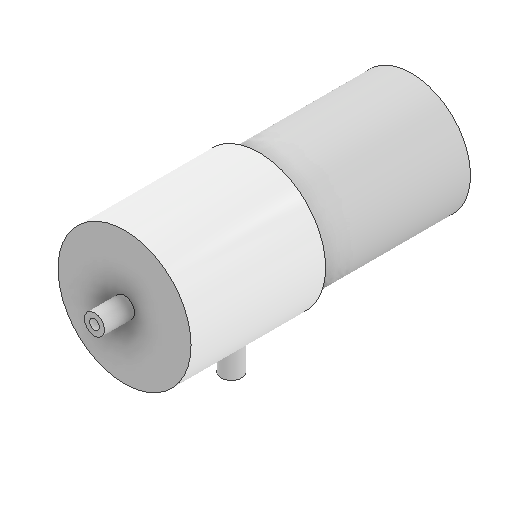
# Autodesk Inventor part: Adafruit_1528_4699_ND
Saved by Autodesk Inventor 2026.2 (Build 302298010, 298A)
## iProperties
Created: 2026-01-21
Part Number: Adafruit_1528_4699_ND
Material: Generic
Document SubType Name: Modeling
Designer: vckot
Density: 1 g/cm^3
Appearance: Default
Author: vckot
Autodesk Inventor part; units mm, degrees
ref_plane "XY Plane" through (0, 0, 0) normal (0, 0, 1) x (1, 0, 0)
sketch "Sketch1" plane through (0, 0, 0) normal (0, 0, 1) x (1, 0, 0)
  circle A0 centre (0, 0) radius 13.5
  circle A1 centre (0, 0) radius 2.05
  circle A2 centre (0, 0) radius 12
  circle A3 centre (0, 0) radius 1
  dimension "d0" = 27
  dimension "d3" = 4.1
  dimension "d6" = 24
  dimension "d20" = 2
  constraints: 4 centre point, 4 coincident
  measures "d0" diameter of A0
  measures "d3" diameter of A1
  measures "d6" diameter of A2
  measures "d20" diameter of A3
extrude "Extrusion1" add sketch "Sketch1" against normal blind 27.3 contours A0 | A1 | A2 | A3
extrude "Extrusion2" add sketch "Sketch1" along normal blind 6.1 contours A1 | A3
extrude "Extrusion3" add sketch "Sketch1" against normal blind 58.2 contours A1 | A2 | A3
ref_plane "Work Plane1" through (0, -13.5, 0) normal (0, 1, 0) x (-1, 0, 0)
sketch "Sketch2" plane through (0, -13.5, 0) normal (0, 1, 0) x (-1, 0, 0)
  circle A0 centre (0, -21.675) radius 2.875
  circle A1 centre (0, -21.675) radius 2.125
  line L0 (13.5, 0) -> (-13.5, 0) projected
  circle A2 centre (0, -21.675) radius 1
  point P0 (0, 0)
  dimension "d10" = 5.75
  dimension "d11" = 21.675
  dimension "d12" = 4.25
  dimension "d17" = 2
  constraints: 3 centre point, 2 coincident
  measures "d10" diameter of A0
  measures "d11" distance from line of A0.centre L0
  measures "d12" diameter of A1
  measures "d17" diameter of A2
extrude "Extrusion4" add sketch "Sketch2" along normal mid plane 4.5 contours A0 | A1 | A2
extrude "Extrusion5" add sketch "Sketch2" against normal blind 8.75 contours A1 | A2
extrude "Extrusion6" cut sketch "Sketch2" against normal through all contours A2
extrude "Extrusion7" cut sketch "Sketch1" along normal through all contours A3
sketch "Sketch3" plane through (0, 0, -58.2) normal (0, 0, -1) x (-1, 0, 0)
  circle A0 centre (0, 0) radius 3.25
  circle A1 centre (0, 0) radius 11.75
  dimension "d23" = 6.5
  dimension "d26" = 23.5
  constraints: 2 centre point, 2 coincident
  measures "d23" diameter of A0
  measures "d26" diameter of A1
extrude "Extrusion9" cut sketch "Sketch3" against normal blind 1
extrude "Extrusion10" add sketch "Sketch3" along normal blind 1.25 contours A0
fillet "Fillet1" radius 0.5 1 edges at (3.25, 0, -59.45)
ref_plane "Work Plane2" through (13.5, 0, 0) normal (1, 0, 0) x (0, 1, 0)
equation "\"d9\" = -0.5 * d0"
body "Solid1"
